Autodesk Fusion 360 part; units mm, degrees
(part 2 of 2)
  spline S18 degree 5 poles (4.156, -4.2818) (4.1594, -4.2853) (4.1663, -4.2922) (4.177, -4.3021) (4.192, -4.3147) (4.2115, -4.3295) (4.2317, -4.3436) (4.2522, -4.3573) (4.273, -4.3707) (4.294, -4.384) (4.3151, -4.3972) (4.3364, -4.4101) (4.358, -4.4227) (4.3799, -4.4349) (4.4021, -4.4468) (4.4246, -4.4584) (4.4473, -4.4697) (4.4702, -4.4807) (4.4933, -4.4916) (4.5165, -4.5022) (4.5399, -4.5126) (4.5635, -4.5228) (4.5873, -4.5328) (4.6112, -4.5425) (4.6354, -4.552) (4.6597, -4.5613) (4.6841, -4.5703) (4.7088, -4.5791) (4.7335, -4.5878) (4.7584, -4.5962) (4.7835, -4.6044) (4.8087, -4.6124) (4.834, -4.6203) (4.8595, -4.6279) (4.8851, -4.6353) (4.9109, -4.6425) (4.9368, -4.6495) (4.9628, -4.6563) (4.9889, -4.6629) (5.0151, -4.6693) (5.0415, -4.6755) (5.068, -4.6816) (5.0946, -4.6874) (5.1213, -4.6931) (5.1481, -4.6985) (5.1751, -4.7038) (5.2021, -4.7088) (5.2293, -4.7137) (5.2566, -4.7184) (5.2839, -4.7229) (5.3114, -4.7272) (5.3389, -4.7314) (5.3666, -4.7353) (5.3944, -4.7391) (5.4222, -4.7426) (5.4502, -4.746) (5.4782, -4.7492) (5.5063, -4.7522) (5.5345, -4.755) (5.5628, -4.7577) (5.5912, -4.7602) (5.6197, -4.7624) (5.6483, -4.7645) (5.6769, -4.7664) (5.7056, -4.7682) (5.7344, -4.7697) (5.7633, -4.7711) (5.7922, -4.7722) (5.8212, -4.7732) (5.8503, -4.774) (5.8795, -4.7747) (5.9029, -4.775) (5.9204, -4.7752) (5.9322, -4.7753) (5.938, -4.7754) knots 0 0 0 0 0 0 0.01428571 0.02857143 0.04285714 0.05714286 0.07142857 0.08571429 0.1 0.11428571 0.12857143 0.14285714 0.15714286 0.17142857 0.18571429 0.2 0.21428571 0.22857143 0.24285714 0.25714286 0.27142857 0.28571429 0.3 0.31428571 0.32857143 0.34285714 0.35714286 0.37142857 0.38571429 0.4 0.41428571 0.42857143 0.44285714 0.45714286 0.47142857 0.48571429 0.5 0.51428571 0.52857143 0.54285714 0.55714286 0.57142857 0.58571429 0.6 0.61428571 0.62857143 0.64285714 0.65714286 0.67142857 0.68571429 0.7 0.71428571 0.72857143 0.74285714 0.75714286 0.77142857 0.78571429 0.8 0.81428571 0.82857143 0.84285714 0.85714286 0.87142857 0.88571429 0.9 0.91428571 0.92857143 0.94285714 0.95714286 0.97142857 0.98571429 1 1 1 1 1 1
  arc A38 (5.938, -4.7754) -> (6.3766, -4.1718) centre (0, 0) ccw
  spline S19 degree 5 poles (6.3766, -4.1718) (6.3747, -4.1662) (6.371, -4.1551) (6.3654, -4.1384) (6.3579, -4.1163) (6.3482, -4.0887) (6.3385, -4.0613) (6.3286, -4.034) (6.3185, -4.0069) (6.3083, -3.9798) (6.2979, -3.9529) (6.2874, -3.9261) (6.2767, -3.8995) (6.2659, -3.873) (6.255, -3.8466) (6.2438, -3.8204) (6.2326, -3.7943) (6.2212, -3.7683) (6.2096, -3.7425) (6.1979, -3.7168) (6.1861, -3.6913) (6.1741, -3.6659) (6.1619, -3.6407) (6.1496, -3.6156) (6.1372, -3.5906) (6.1246, -3.5658) (6.1118, -3.5412) (6.099, -3.5167) (6.0859, -3.4924) (6.0727, -3.4683) (6.0594, -3.4443) (6.0459, -3.4204) (6.0323, -3.3968) (6.0185, -3.3733) (6.0046, -3.3499) (5.9905, -3.3268) (5.9763, -3.3038) (5.962, -3.281) (5.9475, -3.2584) (5.9328, -3.2359) (5.918, -3.2137) (5.903, -3.1916) (5.8879, -3.1697) (5.8727, -3.148) (5.8572, -3.1265) (5.8417, -3.1052) (5.826, -3.0842) (5.8101, -3.0633) (5.7941, -3.0426) (5.7779, -3.0221) (5.7616, -3.0018) (5.7451, -2.9818) (5.7285, -2.9621) (5.7117, -2.9425) (5.6947, -2.9233) (5.6775, -2.9042) (5.6602, -2.8854) (5.6428, -2.8668) (5.6252, -2.8484) (5.6075, -2.8303) (5.5895, -2.8125) (5.5713, -2.7951) (5.5529, -2.778) (5.5343, -2.7614) (5.5154, -2.7451) (5.4964, -2.7291) (5.4773, -2.7133) (5.458, -2.6976) (5.4387, -2.6823) (5.419, -2.6675) (5.3989, -2.6535) (5.3824, -2.6432) (5.3696, -2.6361) (5.3609, -2.6316) (5.3565, -2.6294) knots -1 -1 -1 -1 -1 -1 -0.98571429 -0.97142857 -0.95714286 -0.94285714 -0.92857143 -0.91428571 -0.9 -0.88571429 -0.87142857 -0.85714286 -0.84285714 -0.82857143 -0.81428571 -0.8 -0.78571429 -0.77142857 -0.75714286 -0.74285714 -0.72857143 -0.71428571 -0.7 -0.68571429 -0.67142857 -0.65714286 -0.64285714 -0.62857143 -0.61428571 -0.6 -0.58571429 -0.57142857 -0.55714286 -0.54285714 -0.52857143 -0.51428571 -0.5 -0.48571429 -0.47142857 -0.45714286 -0.44285714 -0.42857143 -0.41428571 -0.4 -0.38571429 -0.37142857 -0.35714286 -0.34285714 -0.32857143 -0.31428571 -0.3 -0.28571429 -0.27142857 -0.25714286 -0.24285714 -0.22857143 -0.21428571 -0.2 -0.18571429 -0.17142857 -0.15714286 -0.14285714 -0.12857143 -0.11428571 -0.1 -0.08571429 -0.07142857 -0.05714286 -0.04285714 -0.02857143 -0.01428571 0 0 0 0 0 0
  line L19 (5.3565, -2.6294) -> (4.5572, -2.2371)
  arc A39 (4.4625, -1.9766) -> (4.5572, -2.2371) centre (4.6453, -2.0576) ccw
  circle A40 centre (0, 0) radius 2.5
  circle A41 centre (0, 0) radius 4
  dimension "d1" = 8
  constraint coincident A0.centre A2.centre
  measures "d1" diameter of A41
extrude "Extrude4" add sketch "Sketch4" along normal blind 3 contours A0 A1 L0 S0 A2 S1 L1 A3 A4 A5 L2 S2 A6 S3 L3 A7 A8 A9 L4 S4 A10 S5 L5 A11 A12 A13 L6 S6 A14 S7 L7 A15 A16 A17 L8 S8 A18 S9 L9 A19 A20 A21 L10 S10 A22 S11 L11 A23 A24 A25 L12 S12 A26 S13 L13 A27 A28 A29 L14 S14 A30 S15 L15 A31 A32 A33 L16 S16 A34 S17 L17 A35 A36 A37 L18 S18 A38 S19 L19 A39
